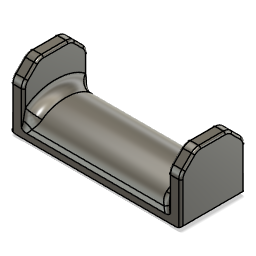
Goalpost_Topper (Autodesk Fusion 360 archive; units mm, degrees)
design "Goalpost Topper Side"
part number: Small
Autodesk Fusion 360 part; units mm, degrees
sketch "Sketch1" plane through (0, 0, 0) normal (0, 0, 1) x (1, 0, 0) in component "Goalpost Topper"
  line L0 (-41, 31) -> (-41, 0)
  line L1 (-41, 0) -> (41, 0)
  line L2 (41, 0) -> (41, 31)
  line L3 (41, 31) -> (35, 31)
  line L4 (35, 2) -> (-35, 2)
  line L5 (-35, 2) -> (-35, 31)
  line L6 (-35, 31) -> (-41, 31)
  line L7 (35, 31) -> (35, 2)
  line L8 (0, 0) -> (0, 2) construction
  dimension "d1" = 29
  dimension "d2" = 70
  dimension "d3" = 6
  dimension "d4" = 2
  dimension "d5" = 29
  constraint vertical L0
  constraint perpendicular L0 L1
  constraint perpendicular L1 L2
  constraint perpendicular L0 L3
  constraint perpendicular L0 L4
  constraint perpendicular L4 L5
  constraint perpendicular L5 L6
  constraint coincident L3.end L7.start
  constraint coincident L8.start origin
  constraint midpoint L4 L8.end
  constraint vertical L8
  constraint perpendicular L4 L7
  constraint coincident L8.start L1
  constraint symmetric L0 L2 L8
  measures "d1" distance of L4.start L3.end
  measures "d2" distance of L4.start L4.end
  measures "d3" distance of L2.end L3.end
  measures "d4" distance of L1 L4
  measures "d5" distance of L4.end L5.end
extrude "Extrude1" add sketch "Sketch1" along normal blind 31 in component "Goalpost Topper"
sketch "Sketch2" plane through (-35, 0, 0) normal (1, 0, 0) x (0, 0, -1) in component "Goalpost Topper"
  line L0 (0, 2) -> (0, 31)
  line L1 (0, 31) -> (-31, 31)
  line L2 (-31, 31) -> (-31, 2)
  line L3 (-31, 2) -> (0, 2)
  line L4 (0, 2) -> (-31, 2)
  ellipse E0 centre (-15.5, 2) end of major axis (0, 2) minor radius 11
  line L5 (-31, 2) -> (0, 2) construction
  line L6 (-15.5, -9) -> (-15.5, 13) construction
  line L7 (-31, 2) -> (0, 2)
  line L8 (0, 0) -> (-31, 0)
  line L9 (0, 2) -> (0, 4)
  line L10 (0, 4) -> (-0.992, 5.872)
  line L11 (-31, 2) -> (-31, 4)
  line L12 (-31, 4) -> (-30.008, 5.872)
  dimension "d47" = 22
  dimension "d99" = 2
  constraint coincident E0 L2.end
  constraint coincident E0 L0.start
  constraint coincident E0 L6.start
  constraint coincident E0 L6.end
  constraint horizontal L5
  constraint coincident L0.start L3.end
  constraint coincident L2.end L3.start
  constraint coincident L0 L9.end
  constraint tangent E0 L9
  constraint coincident E0 L10.end
  constraint coincident L2 L11.end
  constraint tangent E0 L11
  constraint coincident E0 L12.end
  constraint horizontal L9.end L11.end
  constraint horizontal L10.end L12.end
  constraint tangent E0 L10
  measures "d99" distance of L0.start L9.end
extrude "Extrude2" add sketch "Sketch2" along normal up to surface (82 mm away) from surface at -6 contours L0 E0 L9 L10 | L3 L4 E0 L7 | L2 E0 L11 L12 in component "Goalpost Topper"
chamfer "Chamfer7" distance 7.5 angle 45 4 edges at (38, 31, 0) (38, 31, 31) (-38, 31, 0) (-38, 31, 31) in component "Goalpost Topper"
fillet "Fillet7" radius 5 6 edges at (38, 31, 7.5) (38, 31, 23.5) (-38, 31, 7.5) (-38, 31, 23.5) (-38, 23.5, 31) (38, 23.5, 31) in component "Goalpost Topper"
fillet "Fillet7" radius 5 2 edges at (38, 23.5, 0) (-38, 23.5, 0) in component "Goalpost Topper"
chamfer "Chamfer8" distance 1 angle 45 2 edges at (0, 0, 0) (0, 0, 31) in component "Goalpost Topper"
chamfer "Chamfer8" distance 2 angle 45 2 edges at (41, 0, 15.5) (-41, 0, 15.5) in component "Goalpost Topper"
fillet "Fillet3" radius 1 18 edges at (-41, 10.7145, 0) (-41, 23.3423, 0.3806) (-41, 27.25, 3.75) (-41, 30.6194, 7.6577) (-41, 31, 15.5) (-41, 30.6194, 23.3423) (-41, 27.25, 27.25) (-41, 23.3423, 30.6194) (-41, 10.7145, 31) (41, 10.7145, 0) (41, 23.3423, 0.3806) (41, 27.25, 3.75) (41, 30.6194, 7.6577) (41, 31, 15.5) (41, 30.6194, 23.3423) (41, 27.25, 27.25) (41, 23.3423, 30.6194) (41, 10.7145, 31) in component "Goalpost Topper"
fillet "Fillet3" radius 1 18 edges at (35, 12.7145, 0) (35, 23.3423, 0.3806) (35, 27.25, 3.75) (35, 30.6194, 7.6577) (35, 31, 15.5) (35, 30.6194, 23.3423) (35, 27.25, 27.25) (35, 23.3423, 30.6194) (35, 12.7145, 31) (-35, 12.7145, 0) (-35, 23.3423, 0.3806) (-35, 27.25, 3.75) (-35, 30.6194, 7.6577) (-35, 31, 15.5) (-35, 30.6194, 23.3423) (-35, 27.25, 27.25) (-35, 23.3423, 30.6194) (-35, 12.7145, 31) in component "Goalpost Topper"
fillet "Fillet8" radius 5 6 edges at (35, 5.8795, 0.996) (35, 13, 15.5) (35, 5.8795, 30.004) (-35, 5.8795, 30.004) (-35, 13, 15.5) (-35, 5.8795, 0.996) in component "Goalpost Topper"
sketch "Sketch3" plane through (0, 0, 0) normal (0, -1, 0) x (1, 0, 0) in component "Goalpost Topper"
  circle A0 centre (0, 15.5) radius 13
  line L0 (0, 0) -> (0, 30) construction
  line L1 (-54, 15.5) -> (54, 15.5) construction
  line L2 (-39, 1) -> (39, 1)
  line L3 (39, 1) -> (39, 30)
  line L4 (39, 30) -> (-39, 30)
  line L5 (-39, 30) -> (-39, 1)
  dimension "d20" = 26
  constraint coincident L0.start origin
  constraint coincident A0.centre L1
  constraint coincident A0.centre L0
  measures "d20" diameter of A0
extrude "Extrude3" cut sketch "Sketch3" against normal blind 6 contours A0 in component "Goalpost Topper"
thread "Thread1" "ISO Metric profile 28.0 M28x2 6H" major diameter 28.2565 minor diameter 26.0224 pitch 2 angle 60 modelled right hand crest width 0.5434 on face at (12.9838, 4, 14.852) crest through (13.0112, 0.5, 15.5) in component "Goalpost Topper"
sketch "Sketch1 (2)" plane through (-8.9622, 6, -3.7903) normal (0, -1, 0) x (1, 0, 0)
  circle A0 centre (8.9622, 19.2903) radius 9
  spline S0 degree 3 poles (-0.8439, 27.8421) (-1.552, 27.0964) (-2.1691, 26.2693) (-3.2026, 24.4793) (-3.6134, 23.5215) (-4.4022, 20.8568) (-4.5629, 19.1071) (-4.2068, 15.616) (-3.683, 13.9094) (-2.0018, 10.7656) (-0.8514, 9.3638) (1.9406, 7.058) (3.5618, 6.1845) (5.3046, 5.6438) knots -2.761439 -2.761439 -2.761439 -2.761439 -2.452475 -2.452475 -2.140473 -2.140473 -1.617666 -1.617666 -1.08665 -1.08665 -0.547427 -0.547427 0 0 0 0
  arc A1 (5.3046, 5.6438) -> (12.6198, 5.6438) centre (8.9622, 19.2903) ccw
  spline S1 degree 3 poles (12.6198, 5.6438) (13.6765, 5.9716) (14.6909, 6.4226) (16.5836, 7.5488) (17.4564, 8.2181) (19.5235, 10.2334) (20.5512, 11.7201) (21.9633, 14.9806) (22.3436, 16.7186) (22.4111, 20.2152) (22.1081, 21.9397) (20.8633, 25.1481) (19.9433, 26.6046) (18.7683, 27.8421) knots -2.756672 -2.756672 -2.756672 -2.756672 -2.425266 -2.425266 -2.096892 -2.096892 -1.560377 -1.560377 -1.032054 -1.032054 -0.511928 -0.511928 0 0 0 0
  arc A2 (18.7683, 27.8421) -> (-0.8439, 27.8421) centre (8.9622, 19.2903) ccw
  dimension "d26" = 18
  constraint coincident A0.centre A1.centre
  measures "d26" diameter of A0
extrude "Extrude4" cut sketch "Sketch1 (2)" against normal blind 3 contours A0 in component "Goalpost Topper"
ref_plane "WorkPlane1" through (0, 15.5, 15.5) normal (0, 0, -1) x (-1, 0, 0)
sketch "Sketch2 (2)" plane through (0, 0, 15.5) normal (0, 0, -1) x (1, 0, 0)
  line L0 (-9, -6) -> (9, -6)
  line L1 (-7.6706, -9) -> (-9, -6)
  line L2 (-9, -9) -> (-9, -6)
  line L3 (0, -6) -> (0, -9) construction
  line L4 (-9, -9) -> (9, -9)
  constraint coincident L0.start L1.end
  constraint midpoint L0 L3.start
revolve "Revolve1" add sketch "Sketch2 (2)" angle 360 about axis through (0, 6, 15.5) along (0, 1, 0) in component "Goalpost Topper"
fillet "Fillet9" radius 2 4 edges at (-39.5, 0.5, 30.5) (39.5, 0.5, 30.5) (-39.5, 0.5, 0.5) (39.5, 0.5, 0.5) in component "Goalpost Topper"
sketch "Sketch3 (2)" plane through (0, 0, 0) normal (1, 0, 0) x (0, 1, 0)
  line L0 (0, 1.2) -> (0, 3.2)
  line L1 (0, 3.2) -> (2, 3.2)
  line L2 (2, 3.2) -> (0, 1.2)
  line L3 (9, 23.1706) -> (9, 7.8294) construction
  line L4 (9, 15.5) -> (-16, 15.5) construction
  point P0 (9, 23.1706)
  point P1 (9, 7.8294)
  dimension "d106" = 45
  dimension "d107" = 1.2
  dimension "d108" = 2
  dimension "d109" = 25
  constraint vertical L0
  constraint perpendicular L0 L1
  constraint vertical origin L0.start
  constraint coincident P0 L3.start
  constraint coincident P1 L3.end
  constraint midpoint L3 L4.start
  constraint perpendicular L3 L4
  measures "d106" angle of L0 L2
  measures "d107" distance of origin L0.start
  measures "d108" distance of L0.end L1.end
  measures "d109" distance of L4.start L4.end
revolve "Revolve2" cut sketch "Sketch3 (2)" angle 360 about axis through (0, 9, 15.5) along (0, -1, 0) in component "Goalpost Topper"
component "Goalpost Topper" placed x (1, 0, 0) y (0, 1, 0) z (0, 0, 1) at (0, 0, 0)
equation "d1 = Height + 9 mm"
equation "d2 = Width"
equation "d5 = d1"
equation "Height = 20 mm" comment "Zero for no walls. Minimum 15>Bump_Height otherwise"
equation "Width = 70 mm" comment "minmum 27"
equation "Depth = 31 mm" comment "Minimum 31"
equation "d9 = Depth"
equation "Bump_Height = 1 mm"
equation "d47 = Bump_Height * 2 + 20 mm"
equation "Wall_Depth = 15 mm" comment "Maxmum<Depth"
named bodies: "Goalpost_Topper"

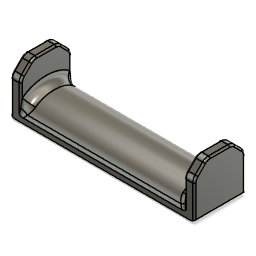
design "Large"
Autodesk Fusion 360 part; units mm, degrees
sketch "Sketch1" plane through (0, 0, 0) normal (0, 0, 1) x (1, 0, 0) in component "Goalpost Topper"
  line L0 (-56, 31) -> (-56, 0)
  line L1 (-56, 0) -> (56, 0)
  line L2 (56, 0) -> (56, 31)
  line L3 (56, 31) -> (50, 31)
  line L4 (50, 2) -> (-50, 2)
  line L5 (-50, 2) -> (-50, 31)
  line L6 (-50, 31) -> (-56, 31)
  line L7 (50, 31) -> (50, 2)
  line L8 (0, 0) -> (0, 2) construction
  dimension "d1" = 29
  dimension "d2" = 100
  dimension "d3" = 6
  dimension "d4" = 2
  dimension "d5" = 29
  constraint vertical L0
  constraint perpendicular L0 L1
  constraint perpendicular L1 L2
  constraint perpendicular L0 L3
  constraint perpendicular L0 L4
  constraint perpendicular L4 L5
  constraint perpendicular L5 L6
  constraint coincident L3.end L7.start
  constraint coincident L8.start origin
  constraint midpoint L4 L8.end
  constraint vertical L8
  constraint perpendicular L4 L7
  constraint coincident L8.start L1
  constraint symmetric L0 L2 L8
  measures "d1" distance of L4.start L3.end
  measures "d2" distance of L4.start L4.end
  measures "d3" distance of L2.end L3.end
  measures "d4" distance of L1 L4
  measures "d5" distance of L4.end L5.end
extrude "Extrude1" add sketch "Sketch1" along normal blind 31 in component "Goalpost Topper"
sketch "Sketch2" plane through (-50, 0, 0) normal (1, 0, 0) x (0, 0, -1) in component "Goalpost Topper"
  line L0 (0, 2) -> (0, 31)
  line L1 (0, 31) -> (-31, 31)
  line L2 (-31, 31) -> (-31, 2)
  line L3 (-31, 2) -> (0, 2)
  line L4 (0, 2) -> (-31, 2)
  ellipse E0 centre (-15.5, 2) end of major axis (0, 2) minor radius 11
  line L5 (-31, 2) -> (0, 2) construction
  line L6 (-15.5, -9) -> (-15.5, 13) construction
  line L7 (-31, 2) -> (0, 2)
  line L8 (0, 0) -> (-31, 0)
  line L9 (0, 2) -> (0, 4)
  line L10 (0, 4) -> (-0.992, 5.872)
  line L11 (-31, 2) -> (-31, 4)
  line L12 (-31, 4) -> (-30.008, 5.872)
  dimension "d47" = 22
  dimension "d99" = 2
  constraint coincident E0 L2.end
  constraint coincident E0 L0.start
  constraint coincident E0 L6.start
  constraint coincident E0 L6.end
  constraint horizontal L5
  constraint coincident L0.start L3.end
  constraint coincident L2.end L3.start
  constraint coincident L0 L9.end
  constraint tangent E0 L9
  constraint coincident E0 L10.end
  constraint coincident L2 L11.end
  constraint tangent E0 L11
  constraint coincident E0 L12.end
  constraint horizontal L9.end L11.end
  constraint horizontal L10.end L12.end
  constraint tangent E0 L10
  measures "d99" distance of L0.start L9.end
extrude "Extrude2" add sketch "Sketch2" along normal up to surface (112 mm away) from surface at -6 contours L0 E0 L9 L10 | L3 L4 E0 L7 | L2 E0 L11 L12 in component "Goalpost Topper"
chamfer "Chamfer7" distance 7.5 angle 45 4 edges at (53, 31, 0) (53, 31, 31) (-53, 31, 0) (-53, 31, 31) in component "Goalpost Topper"
fillet "Fillet7" radius 5 6 edges at (53, 31, 7.5) (53, 31, 23.5) (-53, 31, 7.5) (-53, 31, 23.5) (-53, 23.5, 31) (53, 23.5, 31) in component "Goalpost Topper"
fillet "Fillet7" radius 5 2 edges at (53, 23.5, 0) (-53, 23.5, 0) in component "Goalpost Topper"
chamfer "Chamfer8" distance 1 angle 45 2 edges at (0, 0, 0) (0, 0, 31) in component "Goalpost Topper"
chamfer "Chamfer8" distance 2 angle 45 2 edges at (56, 0, 15.5) (-56, 0, 15.5) in component "Goalpost Topper"
fillet "Fillet3" radius 1 18 edges at (-56, 10.7145, 0) (-56, 23.3423, 0.3806) (-56, 27.25, 3.75) (-56, 30.6194, 7.6577) (-56, 31, 15.5) (-56, 30.6194, 23.3423) (-56, 27.25, 27.25) (-56, 23.3423, 30.6194) (-56, 10.7145, 31) (56, 10.7145, 0) (56, 23.3423, 0.3806) (56, 27.25, 3.75) (56, 30.6194, 7.6577) (56, 31, 15.5) (56, 30.6194, 23.3423) (56, 27.25, 27.25) (56, 23.3423, 30.6194) (56, 10.7145, 31) in component "Goalpost Topper"
fillet "Fillet3" radius 1 18 edges at (50, 12.7145, 0) (50, 23.3423, 0.3806) (50, 27.25, 3.75) (50, 30.6194, 7.6577) (50, 31, 15.5) (50, 30.6194, 23.3423) (50, 27.25, 27.25) (50, 23.3423, 30.6194) (50, 12.7145, 31) (-50, 12.7145, 0) (-50, 23.3423, 0.3806) (-50, 27.25, 3.75) (-50, 30.6194, 7.6577) (-50, 31, 15.5) (-50, 30.6194, 23.3423) (-50, 27.25, 27.25) (-50, 23.3423, 30.6194) (-50, 12.7145, 31) in component "Goalpost Topper"
fillet "Fillet8" radius 5 6 edges at (50, 5.8795, 0.996) (50, 13, 15.5) (50, 5.8795, 30.004) (-50, 5.8795, 30.004) (-50, 13, 15.5) (-50, 5.8795, 0.996) in component "Goalpost Topper"
sketch "Sketch3" plane through (0, 0, 0) normal (0, -1, 0) x (1, 0, 0) in component "Goalpost Topper"
  circle A0 centre (0, 15.5) radius 13
  line L0 (0, 0) -> (0, 30) construction
  line L1 (-54, 15.5) -> (54, 15.5) construction
  line L2 (-54, 1) -> (54, 1)
  line L3 (54, 1) -> (54, 30)
  line L4 (54, 30) -> (-54, 30)
  line L5 (-54, 30) -> (-54, 1)
  dimension "d20" = 26
  constraint coincident L0.start origin
  constraint coincident A0.centre L1
  constraint coincident A0.centre L0
  measures "d20" diameter of A0
extrude "Extrude3" cut sketch "Sketch3" against normal blind 6 contours A0 in component "Goalpost Topper"
thread "Thread1" "ISO Metric profile 28.0 M28x2 6H" major diameter 28.2565 minor diameter 26.0224 pitch 2 angle 60 modelled right hand crest width 0.5434 on face at (12.9838, 4, 14.852) crest through (13.0112, 0.5, 15.5) in component "Goalpost Topper"
sketch "Sketch1 (2)" plane through (-8.9622, 6, -3.7903) normal (0, -1, 0) x (1, 0, 0)
  circle A0 centre (8.9622, 19.2903) radius 9
  spline S0 degree 3 poles (-0.8439, 27.8421) (-1.552, 27.0964) (-2.1691, 26.2693) (-3.2026, 24.4793) (-3.6134, 23.5215) (-4.4022, 20.8568) (-4.5629, 19.1071) (-4.2068, 15.616) (-3.683, 13.9094) (-2.0018, 10.7656) (-0.8514, 9.3638) (1.9406, 7.058) (3.5618, 6.1845) (5.3046, 5.6438) knots -2.761439 -2.761439 -2.761439 -2.761439 -2.452475 -2.452475 -2.140473 -2.140473 -1.617666 -1.617666 -1.08665 -1.08665 -0.547427 -0.547427 0 0 0 0
  arc A1 (5.3046, 5.6438) -> (12.6198, 5.6438) centre (8.9622, 19.2903) ccw
  spline S1 degree 3 poles (12.6198, 5.6438) (13.6765, 5.9716) (14.6909, 6.4226) (16.5836, 7.5488) (17.4564, 8.2181) (19.5235, 10.2334) (20.5512, 11.7201) (21.9633, 14.9806) (22.3436, 16.7186) (22.4111, 20.2152) (22.1081, 21.9397) (20.8633, 25.1481) (19.9433, 26.6046) (18.7683, 27.8421) knots -2.756672 -2.756672 -2.756672 -2.756672 -2.425266 -2.425266 -2.096892 -2.096892 -1.560377 -1.560377 -1.032054 -1.032054 -0.511928 -0.511928 0 0 0 0
  arc A2 (18.7683, 27.8421) -> (-0.8439, 27.8421) centre (8.9622, 19.2903) ccw
  dimension "d26" = 18
  constraint coincident A0.centre A1.centre
  measures "d26" diameter of A0
extrude "Extrude4" cut sketch "Sketch1 (2)" against normal blind 3 contours A0 in component "Goalpost Topper"
ref_plane "WorkPlane1" through (0, 15.5, 15.5) normal (0, 0, -1) x (-1, 0, 0)
sketch "Sketch2 (2)" plane through (0, 0, 15.5) normal (0, 0, -1) x (1, 0, 0)
  line L0 (-9, -6) -> (9, -6)
  line L1 (-7.6706, -9) -> (-9, -6)
  line L2 (-9, -9) -> (-9, -6)
  line L3 (0, -6) -> (0, -9) construction
  line L4 (-9, -9) -> (9, -9)
  constraint coincident L0.start L1.end
  constraint midpoint L0 L3.start
revolve "Revolve1" add sketch "Sketch2 (2)" angle 360 about axis through (0, 6, 15.5) along (0, 1, 0) in component "Goalpost Topper"
fillet "Fillet9" radius 2 4 edges at (-54.5, 0.5, 30.5) (54.5, 0.5, 30.5) (-54.5, 0.5, 0.5) (54.5, 0.5, 0.5) in component "Goalpost Topper"
sketch "Sketch3 (2)" plane through (0, 0, 0) normal (1, 0, 0) x (0, 1, 0)
  line L0 (0, 1.2) -> (0, 3.2)
  line L1 (0, 3.2) -> (2, 3.2)
  line L2 (2, 3.2) -> (0, 1.2)
  line L3 (9, 23.1706) -> (9, 7.8294) construction
  line L4 (9, 15.5) -> (-16, 15.5) construction
  point P0 (9, 23.1706)
  point P1 (9, 7.8294)
  dimension "d106" = 45
  dimension "d107" = 1.2
  dimension "d108" = 2
  dimension "d109" = 25
  constraint vertical L0
  constraint perpendicular L0 L1
  constraint vertical origin L0.start
  constraint coincident P0 L3.start
  constraint coincident P1 L3.end
  constraint midpoint L3 L4.start
  constraint perpendicular L3 L4
  measures "d106" angle of L0 L2
  measures "d107" distance of origin L0.start
  measures "d108" distance of L0.end L1.end
  measures "d109" distance of L4.start L4.end
revolve "Revolve2" cut sketch "Sketch3 (2)" angle 360 about axis through (0, 9, 15.5) along (0, -1, 0) in component "Goalpost Topper"
component "Goalpost Topper" placed x (1, 0, 0) y (0, 1, 0) z (0, 0, 1) at (0, 0, 0)
equation "d1 = Height + 9 mm"
equation "d2 = Width"
equation "d5 = d1"
equation "Height = 20 mm" comment "Zero for no walls. Minimum 15>Bump_Height otherwise"
equation "Width = 100 mm" comment "minmum 27"
equation "Depth = 31 mm" comment "Minimum 31"
equation "d9 = Depth"
equation "Bump_Height = 1 mm"
equation "d47 = Bump_Height * 2 + 20 mm"
equation "Wall_Depth = 20 mm" comment "Maxmum<Depth"
named bodies: "Goalpost_Topper"

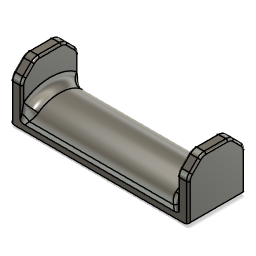
design "Medium"
Autodesk Fusion 360 part; units mm, degrees
sketch "Sketch1" plane through (0, 0, 0) normal (0, 0, 1) x (1, 0, 0) in component "Goalpost Topper"
  line L0 (-48.5, 31) -> (-48.5, 0)
  line L1 (-48.5, 0) -> (48.5, 0)
  line L2 (48.5, 0) -> (48.5, 31)
  line L3 (48.5, 31) -> (42.5, 31)
  line L4 (42.5, 2) -> (-42.5, 2)
  line L5 (-42.5, 2) -> (-42.5, 31)
  line L6 (-42.5, 31) -> (-48.5, 31)
  line L7 (42.5, 31) -> (42.5, 2)
  line L8 (0, 0) -> (0, 2) construction
  dimension "d1" = 29
  dimension "d2" = 85
  dimension "d3" = 6
  dimension "d4" = 2
  dimension "d5" = 29
  constraint vertical L0
  constraint perpendicular L0 L1
  constraint perpendicular L1 L2
  constraint perpendicular L0 L3
  constraint perpendicular L0 L4
  constraint perpendicular L4 L5
  constraint perpendicular L5 L6
  constraint coincident L3.end L7.start
  constraint coincident L8.start origin
  constraint midpoint L4 L8.end
  constraint vertical L8
  constraint perpendicular L4 L7
  constraint coincident L8.start L1
  constraint symmetric L0 L2 L8
  measures "d1" distance of L4.start L3.end
  measures "d2" distance of L4.start L4.end
  measures "d3" distance of L2.end L3.end
  measures "d4" distance of L1 L4
  measures "d5" distance of L4.end L5.end
extrude "Extrude1" add sketch "Sketch1" along normal blind 31 in component "Goalpost Topper"
sketch "Sketch2" plane through (-42.5, 0, 0) normal (1, 0, 0) x (0, 0, -1) in component "Goalpost Topper"
  line L0 (0, 2) -> (0, 31)
  line L1 (0, 31) -> (-31, 31)
  line L2 (-31, 31) -> (-31, 2)
  line L3 (-31, 2) -> (0, 2)
  line L4 (0, 2) -> (-31, 2)
  ellipse E0 centre (-15.5, 2) end of major axis (0, 2) minor radius 11
  line L5 (-31, 2) -> (0, 2) construction
  line L6 (-15.5, -9) -> (-15.5, 13) construction
  line L7 (-31, 2) -> (0, 2)
  line L8 (0, 0) -> (-31, 0)
  line L9 (0, 2) -> (0, 4)
  line L10 (0, 4) -> (-0.992, 5.872)
  line L11 (-31, 2) -> (-31, 4)
  line L12 (-31, 4) -> (-30.008, 5.872)
  dimension "d47" = 22
  dimension "d99" = 2
  constraint coincident E0 L2.end
  constraint coincident E0 L0.start
  constraint coincident E0 L6.start
  constraint coincident E0 L6.end
  constraint horizontal L5
  constraint coincident L0.start L3.end
  constraint coincident L2.end L3.start
  constraint coincident L0 L9.end
  constraint tangent E0 L9
  constraint coincident E0 L10.end
  constraint coincident L2 L11.end
  constraint tangent E0 L11
  constraint coincident E0 L12.end
  constraint horizontal L9.end L11.end
  constraint horizontal L10.end L12.end
  constraint tangent E0 L10
  measures "d99" distance of L0.start L9.end
extrude "Extrude2" add sketch "Sketch2" along normal up to surface (97 mm away) from surface at -6 contours L0 E0 L9 L10 | L3 L4 E0 L7 | L2 E0 L11 L12 in component "Goalpost Topper"
chamfer "Chamfer7" distance 7.5 angle 45 4 edges at (45.5, 31, 0) (45.5, 31, 31) (-45.5, 31, 0) (-45.5, 31, 31) in component "Goalpost Topper"
fillet "Fillet7" radius 5 6 edges at (45.5, 31, 7.5) (45.5, 31, 23.5) (-45.5, 31, 7.5) (-45.5, 31, 23.5) (-45.5, 23.5, 31) (45.5, 23.5, 31) in component "Goalpost Topper"
fillet "Fillet7" radius 5 2 edges at (45.5, 23.5, 0) (-45.5, 23.5, 0) in component "Goalpost Topper"
chamfer "Chamfer8" distance 1 angle 45 2 edges at (0, 0, 0) (0, 0, 31) in component "Goalpost Topper"
chamfer "Chamfer8" distance 2 angle 45 2 edges at (48.5, 0, 15.5) (-48.5, 0, 15.5) in component "Goalpost Topper"
fillet "Fillet3" radius 1 18 edges at (-48.5, 10.7145, 0) (-48.5, 23.3423, 0.3806) (-48.5, 27.25, 3.75) (-48.5, 30.6194, 7.6577) (-48.5, 31, 15.5) (-48.5, 30.6194, 23.3423) (-48.5, 27.25, 27.25) (-48.5, 23.3423, 30.6194) (-48.5, 10.7145, 31) (48.5, 10.7145, 0) (48.5, 23.3423, 0.3806) (48.5, 27.25, 3.75) (48.5, 30.6194, 7.6577) (48.5, 31, 15.5) (48.5, 30.6194, 23.3423) (48.5, 27.25, 27.25) (48.5, 23.3423, 30.6194) (48.5, 10.7145, 31) in component "Goalpost Topper"
fillet "Fillet3" radius 1 18 edges at (42.5, 12.7145, 0) (42.5, 23.3423, 0.3806) (42.5, 27.25, 3.75) (42.5, 30.6194, 7.6577) (42.5, 31, 15.5) (42.5, 30.6194, 23.3423) (42.5, 27.25, 27.25) (42.5, 23.3423, 30.6194) (42.5, 12.7145, 31) (-42.5, 12.7145, 0) (-42.5, 23.3423, 0.3806) (-42.5, 27.25, 3.75) (-42.5, 30.6194, 7.6577) (-42.5, 31, 15.5) (-42.5, 30.6194, 23.3423) (-42.5, 27.25, 27.25) (-42.5, 23.3423, 30.6194) (-42.5, 12.7145, 31) in component "Goalpost Topper"
fillet "Fillet8" radius 5 6 edges at (42.5, 5.8795, 0.996) (42.5, 13, 15.5) (42.5, 5.8795, 30.004) (-42.5, 5.8795, 30.004) (-42.5, 13, 15.5) (-42.5, 5.8795, 0.996) in component "Goalpost Topper"
sketch "Sketch3" plane through (0, 0, 0) normal (0, -1, 0) x (1, 0, 0) in component "Goalpost Topper"
  circle A0 centre (0, 15.5) radius 13
  line L0 (0, 0) -> (0, 30) construction
  line L1 (-54, 15.5) -> (54, 15.5) construction
  line L2 (-46.5, 1) -> (46.5, 1)
  line L3 (46.5, 1) -> (46.5, 30)
  line L4 (46.5, 30) -> (-46.5, 30)
  line L5 (-46.5, 30) -> (-46.5, 1)
  dimension "d20" = 26
  constraint coincident L0.start origin
  constraint coincident A0.centre L1
  constraint coincident A0.centre L0
  measures "d20" diameter of A0
extrude "Extrude3" cut sketch "Sketch3" against normal blind 6 contours A0 in component "Goalpost Topper"
thread "Thread1" "ISO Metric profile 28.0 M28x2 6H" major diameter 28.2565 minor diameter 26.0224 pitch 2 angle 60 modelled right hand crest width 0.5434 on face at (12.9838, 4, 14.852) crest through (13.0112, 0.5, 15.5) in component "Goalpost Topper"
sketch "Sketch1 (2)" plane through (-8.9622, 6, -3.7903) normal (0, -1, 0) x (1, 0, 0)
  circle A0 centre (8.9622, 19.2903) radius 9
  spline S0 degree 3 poles (-0.8439, 27.8421) (-1.552, 27.0964) (-2.1691, 26.2693) (-3.2026, 24.4793) (-3.6134, 23.5215) (-4.4022, 20.8568) (-4.5629, 19.1071) (-4.2068, 15.616) (-3.683, 13.9094) (-2.0018, 10.7656) (-0.8514, 9.3638) (1.9406, 7.058) (3.5618, 6.1845) (5.3046, 5.6438) knots -2.761439 -2.761439 -2.761439 -2.761439 -2.452475 -2.452475 -2.140473 -2.140473 -1.617666 -1.617666 -1.08665 -1.08665 -0.547427 -0.547427 0 0 0 0
  arc A1 (5.3046, 5.6438) -> (12.6198, 5.6438) centre (8.9622, 19.2903) ccw
  spline S1 degree 3 poles (12.6198, 5.6438) (13.6765, 5.9716) (14.6909, 6.4226) (16.5836, 7.5488) (17.4564, 8.2181) (19.5235, 10.2334) (20.5512, 11.7201) (21.9633, 14.9806) (22.3436, 16.7186) (22.4111, 20.2152) (22.1081, 21.9397) (20.8633, 25.1481) (19.9433, 26.6046) (18.7683, 27.8421) knots -2.756672 -2.756672 -2.756672 -2.756672 -2.425266 -2.425266 -2.096892 -2.096892 -1.560377 -1.560377 -1.032054 -1.032054 -0.511928 -0.511928 0 0 0 0
  arc A2 (18.7683, 27.8421) -> (-0.8439, 27.8421) centre (8.9622, 19.2903) ccw
  dimension "d26" = 18
  constraint coincident A0.centre A1.centre
  measures "d26" diameter of A0
extrude "Extrude4" cut sketch "Sketch1 (2)" against normal blind 3 contours A0 in component "Goalpost Topper"
ref_plane "WorkPlane1" through (0, 15.5, 15.5) normal (0, 0, -1) x (-1, 0, 0)
sketch "Sketch2 (2)" plane through (0, 0, 15.5) normal (0, 0, -1) x (1, 0, 0)
  line L0 (-9, -6) -> (9, -6)
  line L1 (-7.6706, -9) -> (-9, -6)
  line L2 (-9, -9) -> (-9, -6)
  line L3 (0, -6) -> (0, -9) construction
  line L4 (-9, -9) -> (9, -9)
  constraint coincident L0.start L1.end
  constraint midpoint L0 L3.start
revolve "Revolve1" add sketch "Sketch2 (2)" angle 360 about axis through (0, 6, 15.5) along (0, 1, 0) in component "Goalpost Topper"
fillet "Fillet9" radius 2 4 edges at (-47, 0.5, 30.5) (47, 0.5, 30.5) (-47, 0.5, 0.5) (47, 0.5, 0.5) in component "Goalpost Topper"
sketch "Sketch3 (2)" plane through (0, 0, 0) normal (1, 0, 0) x (0, 1, 0)
  line L0 (0, 1.2) -> (0, 3.2)
  line L1 (0, 3.2) -> (2, 3.2)
  line L2 (2, 3.2) -> (0, 1.2)
  line L3 (9, 23.1706) -> (9, 7.8294) construction
  line L4 (9, 15.5) -> (-16, 15.5) construction
  point P0 (9, 23.1706)
  point P1 (9, 7.8294)
  dimension "d106" = 45
  dimension "d107" = 1.2
  dimension "d108" = 2
  dimension "d109" = 25
  constraint vertical L0
  constraint perpendicular L0 L1
  constraint vertical origin L0.start
  constraint coincident P0 L3.start
  constraint coincident P1 L3.end
  constraint midpoint L3 L4.start
  constraint perpendicular L3 L4
  measures "d106" angle of L0 L2
  measures "d107" distance of origin L0.start
  measures "d108" distance of L0.end L1.end
  measures "d109" distance of L4.start L4.end
revolve "Revolve2" cut sketch "Sketch3 (2)" angle 360 about axis through (0, 9, 15.5) along (0, -1, 0) in component "Goalpost Topper"
component "Goalpost Topper" placed x (1, 0, 0) y (0, 1, 0) z (0, 0, 1) at (0, 0, 0)
equation "d1 = Height + 9 mm"
equation "d2 = Width"
equation "d5 = d1"
equation "Height = 20 mm" comment "Zero for no walls. Minimum 15>Bump_Height otherwise"
equation "Width = 85 mm" comment "minmum 27"
equation "Depth = 31 mm" comment "Minimum 31"
equation "d9 = Depth"
equation "Bump_Height = 1 mm"
equation "d47 = Bump_Height * 2 + 20 mm"
equation "Wall_Depth = 18 mm" comment "Maxmum<Depth"
named bodies: "Goalpost_Topper"

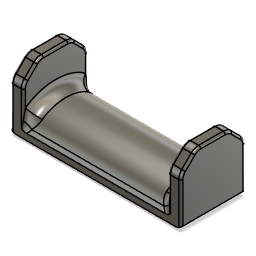
design "Small"
Autodesk Fusion 360 part; units mm, degrees
sketch "Sketch1" plane through (0, 0, 0) normal (0, 0, 1) x (1, 0, 0) in component "Goalpost Topper"
  line L0 (-41, 31) -> (-41, 0)
  line L1 (-41, 0) -> (41, 0)
  line L2 (41, 0) -> (41, 31)
  line L3 (41, 31) -> (35, 31)
  line L4 (35, 2) -> (-35, 2)
  line L5 (-35, 2) -> (-35, 31)
  line L6 (-35, 31) -> (-41, 31)
  line L7 (35, 31) -> (35, 2)
  line L8 (0, 0) -> (0, 2) construction
  dimension "d1" = 29
  dimension "d2" = 70
  dimension "d3" = 6
  dimension "d4" = 2
  dimension "d5" = 29
  constraint vertical L0
  constraint perpendicular L0 L1
  constraint perpendicular L1 L2
  constraint perpendicular L0 L3
  constraint perpendicular L0 L4
  constraint perpendicular L4 L5
  constraint perpendicular L5 L6
  constraint coincident L3.end L7.start
  constraint coincident L8.start origin
  constraint midpoint L4 L8.end
  constraint vertical L8
  constraint perpendicular L4 L7
  constraint coincident L8.start L1
  constraint symmetric L0 L2 L8
  measures "d1" distance of L4.start L3.end
  measures "d2" distance of L4.start L4.end
  measures "d3" distance of L2.end L3.end
  measures "d4" distance of L1 L4
  measures "d5" distance of L4.end L5.end
extrude "Extrude1" add sketch "Sketch1" along normal blind 31 in component "Goalpost Topper"
sketch "Sketch2" plane through (-35, 0, 0) normal (1, 0, 0) x (0, 0, -1) in component "Goalpost Topper"
  line L0 (0, 2) -> (0, 31)
  line L1 (0, 31) -> (-31, 31)
  line L2 (-31, 31) -> (-31, 2)
  line L3 (-31, 2) -> (0, 2)
  line L4 (0, 2) -> (-31, 2)
  ellipse E0 centre (-15.5, 2) end of major axis (0, 2) minor radius 11
  line L5 (-31, 2) -> (0, 2) construction
  line L6 (-15.5, -9) -> (-15.5, 13) construction
  line L7 (-31, 2) -> (0, 2)
  line L8 (0, 0) -> (-31, 0)
  line L9 (0, 2) -> (0, 4)
  line L10 (0, 4) -> (-0.992, 5.872)
  line L11 (-31, 2) -> (-31, 4)
  line L12 (-31, 4) -> (-30.008, 5.872)
  dimension "d47" = 22
  dimension "d99" = 2
  constraint coincident E0 L2.end
  constraint coincident E0 L0.start
  constraint coincident E0 L6.start
  constraint coincident E0 L6.end
  constraint horizontal L5
  constraint coincident L0.start L3.end
  constraint coincident L2.end L3.start
  constraint coincident L0 L9.end
  constraint tangent E0 L9
  constraint coincident E0 L10.end
  constraint coincident L2 L11.end
  constraint tangent E0 L11
  constraint coincident E0 L12.end
  constraint horizontal L9.end L11.end
  constraint horizontal L10.end L12.end
  constraint tangent E0 L10
  measures "d99" distance of L0.start L9.end
extrude "Extrude2" add sketch "Sketch2" along normal up to surface (82 mm away) from surface at -6 contours L0 E0 L9 L10 | L3 L4 E0 L7 | L2 E0 L11 L12 in component "Goalpost Topper"
chamfer "Chamfer7" distance 7.5 angle 45 4 edges at (38, 31, 0) (38, 31, 31) (-38, 31, 0) (-38, 31, 31) in component "Goalpost Topper"
fillet "Fillet7" radius 5 6 edges at (38, 31, 7.5) (38, 31, 23.5) (-38, 31, 7.5) (-38, 31, 23.5) (-38, 23.5, 31) (38, 23.5, 31) in component "Goalpost Topper"
fillet "Fillet7" radius 5 2 edges at (38, 23.5, 0) (-38, 23.5, 0) in component "Goalpost Topper"
chamfer "Chamfer8" distance 1 angle 45 2 edges at (0, 0, 0) (0, 0, 31) in component "Goalpost Topper"
chamfer "Chamfer8" distance 2 angle 45 2 edges at (41, 0, 15.5) (-41, 0, 15.5) in component "Goalpost Topper"
fillet "Fillet3" radius 1 18 edges at (-41, 10.7145, 0) (-41, 23.3423, 0.3806) (-41, 27.25, 3.75) (-41, 30.6194, 7.6577) (-41, 31, 15.5) (-41, 30.6194, 23.3423) (-41, 27.25, 27.25) (-41, 23.3423, 30.6194) (-41, 10.7145, 31) (41, 10.7145, 0) (41, 23.3423, 0.3806) (41, 27.25, 3.75) (41, 30.6194, 7.6577) (41, 31, 15.5) (41, 30.6194, 23.3423) (41, 27.25, 27.25) (41, 23.3423, 30.6194) (41, 10.7145, 31) in component "Goalpost Topper"
fillet "Fillet3" radius 1 18 edges at (35, 12.7145, 0) (35, 23.3423, 0.3806) (35, 27.25, 3.75) (35, 30.6194, 7.6577) (35, 31, 15.5) (35, 30.6194, 23.3423) (35, 27.25, 27.25) (35, 23.3423, 30.6194) (35, 12.7145, 31) (-35, 12.7145, 0) (-35, 23.3423, 0.3806) (-35, 27.25, 3.75) (-35, 30.6194, 7.6577) (-35, 31, 15.5) (-35, 30.6194, 23.3423) (-35, 27.25, 27.25) (-35, 23.3423, 30.6194) (-35, 12.7145, 31) in component "Goalpost Topper"
fillet "Fillet8" radius 5 6 edges at (35, 5.8795, 0.996) (35, 13, 15.5) (35, 5.8795, 30.004) (-35, 5.8795, 30.004) (-35, 13, 15.5) (-35, 5.8795, 0.996) in component "Goalpost Topper"
sketch "Sketch3" plane through (0, 0, 0) normal (0, -1, 0) x (1, 0, 0) in component "Goalpost Topper"
  circle A0 centre (0, 15.5) radius 13
  line L0 (0, 0) -> (0, 30) construction
  line L1 (-54, 15.5) -> (54, 15.5) construction
  line L2 (-39, 1) -> (39, 1)
  line L3 (39, 1) -> (39, 30)
  line L4 (39, 30) -> (-39, 30)
  line L5 (-39, 30) -> (-39, 1)
  dimension "d20" = 26
  constraint coincident L0.start origin
  constraint coincident A0.centre L1
  constraint coincident A0.centre L0
  measures "d20" diameter of A0
extrude "Extrude3" cut sketch "Sketch3" against normal blind 6 contours A0 in component "Goalpost Topper"
thread "Thread1" "ISO Metric profile 28.0 M28x2 6H" major diameter 28.2565 minor diameter 26.0224 pitch 2 angle 60 modelled right hand crest width 0.5434 on face at (12.9838, 4, 14.852) crest through (13.0112, 0.5, 15.5) in component "Goalpost Topper"
sketch "Sketch1 (2)" plane through (-8.9622, 6, -3.7903) normal (0, -1, 0) x (1, 0, 0)
  circle A0 centre (8.9622, 19.2903) radius 9
  spline S0 degree 3 poles (-0.8439, 27.8421) (-1.552, 27.0964) (-2.1691, 26.2693) (-3.2026, 24.4793) (-3.6134, 23.5215) (-4.4022, 20.8568) (-4.5629, 19.1071) (-4.2068, 15.616) (-3.683, 13.9094) (-2.0018, 10.7656) (-0.8514, 9.3638) (1.9406, 7.058) (3.5618, 6.1845) (5.3046, 5.6438) knots -2.761439 -2.761439 -2.761439 -2.761439 -2.452475 -2.452475 -2.140473 -2.140473 -1.617666 -1.617666 -1.08665 -1.08665 -0.547427 -0.547427 0 0 0 0
  arc A1 (5.3046, 5.6438) -> (12.6198, 5.6438) centre (8.9622, 19.2903) ccw
  spline S1 degree 3 poles (12.6198, 5.6438) (13.6765, 5.9716) (14.6909, 6.4226) (16.5836, 7.5488) (17.4564, 8.2181) (19.5235, 10.2334) (20.5512, 11.7201) (21.9633, 14.9806) (22.3436, 16.7186) (22.4111, 20.2152) (22.1081, 21.9397) (20.8633, 25.1481) (19.9433, 26.6046) (18.7683, 27.8421) knots -2.756672 -2.756672 -2.756672 -2.756672 -2.425266 -2.425266 -2.096892 -2.096892 -1.560377 -1.560377 -1.032054 -1.032054 -0.511928 -0.511928 0 0 0 0
  arc A2 (18.7683, 27.8421) -> (-0.8439, 27.8421) centre (8.9622, 19.2903) ccw
  dimension "d26" = 18
  constraint coincident A0.centre A1.centre
  measures "d26" diameter of A0
extrude "Extrude4" cut sketch "Sketch1 (2)" against normal blind 3 contours A0 in component "Goalpost Topper"
ref_plane "WorkPlane1" through (0, 15.5, 15.5) normal (0, 0, -1) x (-1, 0, 0)
sketch "Sketch2 (2)" plane through (0, 0, 15.5) normal (0, 0, -1) x (1, 0, 0)
  line L0 (-9, -6) -> (9, -6)
  line L1 (-7.6706, -9) -> (-9, -6)
  line L2 (-9, -9) -> (-9, -6)
  line L3 (0, -6) -> (0, -9) construction
  line L4 (-9, -9) -> (9, -9)
  constraint coincident L0.start L1.end
  constraint midpoint L0 L3.start
revolve "Revolve1" add sketch "Sketch2 (2)" angle 360 about axis through (0, 6, 15.5) along (0, 1, 0) in component "Goalpost Topper"
fillet "Fillet9" radius 2 4 edges at (-39.5, 0.5, 30.5) (39.5, 0.5, 30.5) (-39.5, 0.5, 0.5) (39.5, 0.5, 0.5) in component "Goalpost Topper"
sketch "Sketch3 (2)" plane through (0, 0, 0) normal (1, 0, 0) x (0, 1, 0)
  line L0 (0, 1.2) -> (0, 3.2)
  line L1 (0, 3.2) -> (2, 3.2)
  line L2 (2, 3.2) -> (0, 1.2)
  line L3 (9, 23.1706) -> (9, 7.8294) construction
  line L4 (9, 15.5) -> (-16, 15.5) construction
  point P0 (9, 23.1706)
  point P1 (9, 7.8294)
  dimension "d106" = 45
  dimension "d107" = 1.2
  dimension "d108" = 2
  dimension "d109" = 25
  constraint vertical L0
  constraint perpendicular L0 L1
  constraint vertical origin L0.start
  constraint coincident P0 L3.start
  constraint coincident P1 L3.end
  constraint midpoint L3 L4.start
  constraint perpendicular L3 L4
  measures "d106" angle of L0 L2
  measures "d107" distance of origin L0.start
  measures "d108" distance of L0.end L1.end
  measures "d109" distance of L4.start L4.end
revolve "Revolve2" cut sketch "Sketch3 (2)" angle 360 about axis through (0, 9, 15.5) along (0, -1, 0) in component "Goalpost Topper"
component "Goalpost Topper" placed x (1, 0, 0) y (0, 1, 0) z (0, 0, 1) at (0, 0, 0)
equation "d1 = Height + 9 mm"
equation "d2 = Width"
equation "d5 = d1"
equation "Height = 20 mm" comment "Zero for no walls. Minimum 15>Bump_Height otherwise"
equation "Width = 70 mm" comment "minmum 27"
equation "Depth = 31 mm" comment "Minimum 31"
equation "d9 = Depth"
equation "Bump_Height = 1 mm"
equation "d47 = Bump_Height * 2 + 20 mm"
equation "Wall_Depth = 15 mm" comment "Maxmum<Depth"
named bodies: "Goalpost_Topper"
